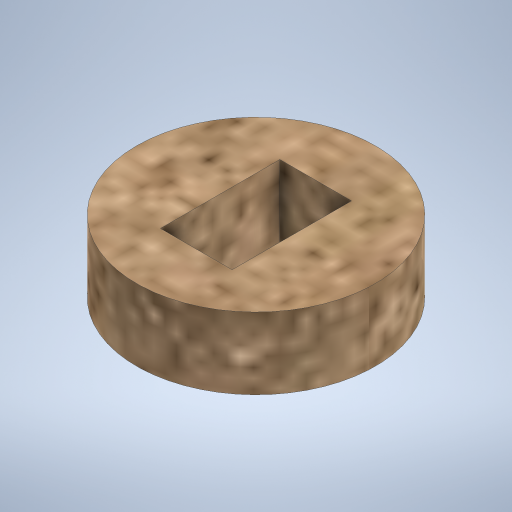
# Autodesk Inventor part: Camera_Support
Saved by Autodesk Inventor 2024 (Build 280153000, 153)
## iProperties
Created: 2023-11-23
Part Number: Camera_Support
Material: MDF Tablero de fibras de densidad media
Document SubType Name: Modeling
Designer: marco
Density: 0.8 g/cm^3
Appearance: Cartón - Ondulado
Author: marco
Autodesk Inventor part; units mm, degrees
ref_plane "YZ Plane" through (0, 0, 0) normal (1, 0, 0) x (0, 1, 0)
ref_plane "XZ Plane" through (0, 0, 0) normal (0, 1, 0) x (-1, 0, 0)
ref_plane "XY Plane" through (0, 0, 0) normal (0, 0, 1) x (1, 0, 0)
sketch "Boceto2" plane through (0, 0, 0) normal (0, 1, 0) x (-1, 0, 0)
  circle A0 centre (0, 0) radius 5
  line L0 (1.5, -2.5) -> (-1.5, -2.5)
  line L1 (-1.5, -2.5) -> (-1.5, 2.5)
  line L2 (-1.5, 2.5) -> (1.5, 2.5)
  line L3 (1.5, 2.5) -> (1.5, -2.5)
  point P0 (-1.5, -2.5)
  constraints: 8 end point, 1 centre point, 1 vertical
extrude "Extrusión1" add sketch "Boceto2" along normal blind 3
